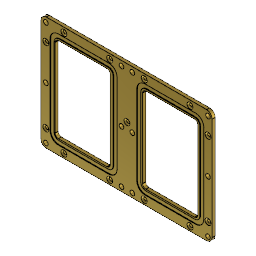
1006351A-exact-GASKET (Autodesk Fusion 360 design; units mm, degrees)
Autodesk Fusion 360 part; units mm, degrees
sketch "Front-OuterDimensionsAndHoles" plane through (0, 0, 0) normal (0, 1, 0) x (1, 0, 0) in component "1006351A-GASKET"
  line L0 (-137.0277, -51.6717) -> (147.7462, -51.6717) construction
  line L1 (-113.1932, -37.4477) -> (126.9355, -37.4477) construction
  line L2 (-111.6736, 46.3723) -> (88.9542, 46.3723) construction
  line L3 (-83.38, 4.4623) -> (113.9408, 4.4623) construction
  line L4 (77.012, -30.3357) -> (138.7437, -30.3357) construction
  line L5 (77.3795, 43.3243) -> (102.1824, 43.3243) construction
  line L6 (-79.2352, -152.4901) -> (-79.2352, 67.7682) construction
  line L7 (80.7848, -152.4901) -> (80.7848, 99.4049) construction
  line L8 (-16.2432, -127.3246) -> (-16.2432, -37.4477) construction
  line L9 (-61.4552, -139.7875) -> (-61.4552, -23.5467) construction
  line L10 (-4.5592, -114.8617) -> (-4.5592, -39.3651) construction
  line L11 (0.7748, -102.6384) -> (0.7748, 79.7518) construction
  line L12 (6.1088, -89.6961) -> (6.1088, 17.4372) construction
  line L13 (122.5447, -1.8877) -> (-114.7303, -1.8877) construction
  line L14 (151.0657, 56.0243) -> (-121.6808, 56.0243) construction
  line L15 (-84.366, -162.1054) -> (-84.366, 89.1529) construction
  line L16 (84.8488, -151.7017) -> (84.8488, 106.4269) construction
  line L17 (17.7928, -77.6983) -> (17.7928, -42.3651) construction
  line L18 (63.0048, -65.3317) -> (63.0048, -43.9355) construction
  line L19 (-137.1695, 60.5963) -> (174.7441, 60.5963) construction
  line L20 (-87.8994, -47.0997) -> (156.6849, -47.0997) construction
  line L21 (70.6248, 70.8097) -> (70.6248, -45.2683) construction
  line L22 (16.2688, 71.2679) -> (16.2688, -42.3651) construction
  line L23 (-15.786, 70.5042) -> (-15.786, -42.9773) construction
  line L24 (-70.142, 108.0768) -> (-70.142, -44.9628) construction
  line L25 (-10.9092, 93.2616) -> (-10.9092, -44.6574) construction
  line L26 (73.9383, 85.014) -> (73.9383, -42.8245) construction
  line L27 (-101.4005, 49.5796) -> (76.5348, 49.5796) construction
  line L28 (-100.0259, -41.454) -> (76.8403, -41.454) construction
  line L29 (-78.8288, -51.9257) -> (79.3116, -51.9257)
  line L30 (84.8488, -46.3885) -> (84.8488, 54.8051)
  line L31 (79.3116, 60.3423) -> (-78.8288, 60.3423)
  line L32 (-84.366, 54.8051) -> (-84.366, -46.3885)
  line L33 (-66.967, -37.7017) -> (-18.961, -37.7017)
  line L34 (-15.786, -34.5267) -> (-15.786, 42.9433)
  line L35 (-18.961, 46.1183) -> (-66.967, 46.1183)
  line L36 (-70.142, 42.9433) -> (-70.142, -34.5267)
  line L37 (19.4438, -37.7017) -> (67.4498, -37.7017)
  line L38 (70.6248, -34.5267) -> (70.6248, 42.9433)
  line L39 (67.4498, 46.1183) -> (19.4438, 46.1183)
  line L40 (16.2688, 42.9433) -> (16.2688, -34.5267)
  arc A0 (-84.366, -46.3885) -> (-78.8288, -51.9257) centre (-78.8288, -46.3885) ccw
  arc A1 (-78.8288, 60.3423) -> (-84.366, 54.8051) centre (-78.8288, 54.8051) ccw
  arc A2 (84.8488, 54.8051) -> (79.3116, 60.3423) centre (79.3116, 54.8051) ccw
  arc A3 (-70.142, -34.5267) -> (-66.967, -37.7017) centre (-66.967, -34.5267) ccw
  arc A4 (-18.961, -37.7017) -> (-15.786, -34.5267) centre (-18.961, -34.5267) ccw
  arc A5 (-15.786, 42.9433) -> (-18.961, 46.1183) centre (-18.961, 42.9433) ccw
  arc A6 (-66.967, 46.1183) -> (-70.142, 42.9433) centre (-66.967, 42.9433) ccw
  arc A7 (67.4498, -37.7017) -> (70.6248, -34.5267) centre (67.4498, -34.5267) ccw
  arc A8 (70.6248, 42.9433) -> (67.4498, 46.1183) centre (67.4498, 42.9433) ccw
  arc A9 (19.4438, 46.1183) -> (16.2688, 42.9433) centre (19.4438, 42.9433) ccw
  arc A10 (16.2688, -34.5267) -> (19.4438, -37.7017) centre (19.4438, -34.5267) ccw
  arc A11 (79.3116, -51.9257) -> (84.8488, -46.3885) centre (79.3116, -46.3885) ccw
  line L41 (-100.3246, -43.4352) -> (86.6573, -43.4352) construction
  line L42 (-99.9078, -39.4728) -> (77.154, -39.4728) construction
  line L43 (-94.8446, 47.5984) -> (76.1721, 47.5984) construction
  line L44 (-94.4522, 51.5608) -> (76.1721, 51.5608) construction
  line L45 (-73.1392, 86.7279) -> (-73.1392, -45.4577) construction
  line L46 (-8.928, 72.5566) -> (-8.928, -44.6167) construction
  line L47 (-12.8904, 72.2199) -> (-12.8904, -44.6167) construction
  line L48 (-75.1204, 70.9572) -> (-75.1204, -44.6167) construction
  line L49 (-71.158, 71.0414) -> (-71.158, -44.3641) construction
  line L50 (-66.967, 51.5608) -> (-17.0814, 51.5608)
  line L51 (-8.928, 43.4074) -> (-8.928, -35.2818)
  line L52 (-17.0814, -43.4352) -> (-66.967, -43.4352)
  line L53 (-75.1204, -35.2818) -> (-75.1204, 43.4074)
  line L54 (-66.205, 47.5984) -> (-17.8434, 47.5984)
  line L55 (-12.8904, 42.6454) -> (-12.8904, -34.5198)
  line L56 (-17.8434, -39.4728) -> (-66.205, -39.4728)
  line L57 (-71.158, -34.5198) -> (-71.158, 42.6454)
  arc A12 (-75.1204, -35.2818) -> (-66.967, -43.4352) centre (-66.967, -35.2818) ccw
  arc A13 (-17.0814, -43.4352) -> (-8.928, -35.2818) centre (-17.0814, -35.2818) ccw
  arc A14 (-8.928, 43.4074) -> (-17.0814, 51.5608) centre (-17.0814, 43.4074) ccw
  arc A15 (-66.967, 51.5608) -> (-75.1204, 43.4074) centre (-66.967, 43.4074) ccw
  arc A16 (-71.158, -34.5198) -> (-66.205, -39.4728) centre (-66.205, -34.5198) ccw
  arc A17 (-66.205, 47.5984) -> (-71.158, 42.6454) centre (-66.205, 42.6454) ccw
  arc A18 (-12.8904, 42.6454) -> (-17.8434, 47.5984) centre (-17.8434, 42.6454) ccw
  arc A19 (-17.8434, -39.4728) -> (-12.8904, -34.5198) centre (-17.8434, -34.5198) ccw
  line L58 (18.631, -43.4352) -> (68.5166, -43.4352)
  arc A20 (68.5166, -43.4352) -> (76.67, -35.2818) centre (68.5166, -35.2818) ccw
  line L59 (76.67, -35.2818) -> (76.67, 43.4074)
  arc A21 (76.67, 43.4074) -> (68.5166, 51.5608) centre (68.5166, 43.4074) ccw
  line L60 (68.5166, 51.5608) -> (18.631, 51.5608)
  arc A22 (18.631, 51.5608) -> (10.4776, 43.4074) centre (18.631, 43.4074) ccw
  line L61 (10.4776, 43.4074) -> (10.4776, -35.2818)
  arc A23 (10.4776, -35.2818) -> (18.631, -43.4352) centre (18.631, -35.2818) ccw
  line L62 (19.393, -39.4728) -> (67.7546, -39.4728)
  arc A24 (67.7546, -39.4728) -> (72.7076, -34.5198) centre (67.7546, -34.5198) ccw
  line L63 (72.7076, -34.5198) -> (72.7076, 42.6454)
  arc A25 (72.7076, 42.6454) -> (67.7546, 47.5984) centre (67.7546, 42.6454) ccw
  line L64 (67.7546, 47.5984) -> (19.393, 47.5984)
  arc A26 (19.393, 47.5984) -> (14.44, 42.6454) centre (19.393, 42.6454) ccw
  line L65 (14.44, 42.6454) -> (14.44, -34.5198)
  line L66 (101.4573, -39.4728) -> (-75.6045, -39.4728) construction
  arc A27 (14.44, -34.5198) -> (19.393, -39.4728) centre (19.393, -34.5198) ccw
  point P0 (-79.2352, -47.0997)
  point P1 (-4.5592, -47.0997)
  point P2 (6.1088, -47.0997)
  point P3 (80.7848, -47.0997)
  point P4 (80.7848, 4.4623)
  point P5 (6.1088, 4.4623)
  point P6 (-79.2352, 4.4623)
  point P7 (-4.5592, 4.4623)
  point P8 (80.7848, 56.0243)
  point P9 (6.1088, 56.0243)
  point P10 (-4.5592, 56.0243)
  point P11 (-79.2352, 56.0243)
  point P12 (80.7848, -30.3357)
  point P13 (80.7848, 43.3243)
  point P14 (63.0048, -47.0997)
  point P15 (17.7928, -47.0997)
  point P16 (17.7928, 56.0243)
  point P17 (63.0048, 56.0243)
  point P18 (0.7748, -1.8877)
  point P19 (-16.2432, -47.0997)
  point P20 (-61.4552, -47.0997)
  point P21 (-79.2352, -30.3357)
  point P22 (-79.2352, 43.3243)
  point P23 (-61.4552, 56.0243)
  point P24 (-16.2432, 56.0243)
  dimension "d1" = 169.2148
  dimension "d2" = 4.064
  dimension "d3" = 160.02
  dimension "d4" = 142.24
  dimension "d5" = 97.028
  dimension "d6" = 85.344
  dimension "d7" = 80.01
  dimension "d8" = 74.676
  dimension "d9" = 17.78
  dimension "d10" = 62.992
  dimension "d12" = 112.268
  dimension "d13" = 103.124
  dimension "d14" = 51.562
  dimension "d16" = 57.912
  dimension "d17" = 86.36
  dimension "d18" = 12.7
  dimension "d19" = 14.224
  dimension "d20" = 4.572
  dimension "d21" = 14.224
  dimension "d22" = 14.224
  dimension "d23" = 54.356
  dimension "d24" = 54.356
  dimension "d25" = 91.0336
  dimension "d26" = 14.224
  dimension "d27" = 5.5372
  dimension "d28" = 5.5372
  dimension "d29" = 5.5372
  dimension "d30" = 3.175
  dimension "d31" = 3.175
  dimension "d32" = 3.175
  dimension "d33" = 3.175
  dimension "d34" = 3.175
  dimension "d35" = 3.175
  dimension "d36" = 3.175
  dimension "d37" = 3.175
  dimension "d40" = 5.5372
  dimension "d49" = 1.9812
  dimension "d50" = 1.9812
  dimension "d51" = 1.9812
  dimension "d52" = 1.9812
  dimension "d53" = 91.694
  dimension "d54" = 62.23
  dimension "d55" = 1.9812
  dimension "d56" = 1.9812
  dimension "d57" = 1.9812
  dimension "d58" = 1.9812
  dimension "d59" = 8.1534
  dimension "d60" = 8.1534
  dimension "d61" = 8.1534
  dimension "d62" = 8.1534
  dimension "d63" = 4.953
  dimension "d64" = 4.953
  dimension "d65" = 4.953
  dimension "d66" = 4.953
  constraint horizontal L0
  constraint horizontal L1
  constraint parallel L1 L2
  constraint horizontal L3
  constraint parallel L1 L4
  constraint horizontal L5
  constraint perpendicular L0 L6
  constraint perpendicular L2 L7
  constraint coincident L1 L8.end
  constraint perpendicular L1 L8
  constraint vertical L9
  constraint perpendicular L0 L10
  constraint perpendicular L2 L11
  constraint perpendicular L3 L12
  constraint perpendicular L12 L13
  constraint parallel L2 L14
  constraint perpendicular L14 L15
  constraint perpendicular L14 L16
  constraint perpendicular L0 L17
  constraint perpendicular L0 L18
  constraint horizontal L19
  constraint perpendicular L15 L20
  constraint perpendicular L1 L21
  constraint perpendicular L1 L22
  constraint perpendicular L20 L23
  constraint perpendicular L1 L24
  constraint perpendicular L1 L25
  constraint perpendicular L1 L26
  constraint perpendicular L26 L27
  constraint perpendicular L26 L28
  constraint horizontal L29
  constraint vertical L30
  constraint horizontal L31
  constraint vertical L32
  constraint horizontal L33
  constraint vertical L34
  constraint horizontal L35
  constraint vertical L36
  constraint horizontal L37
  constraint vertical L38
  constraint horizontal L39
  constraint vertical L40
  constraint tangent L29 A0
  constraint tangent L32 A0
  constraint tangent L32 A1
  constraint tangent L31 A1
  constraint tangent L31 A2
  constraint tangent L30 A2
  constraint tangent L33 A3
  constraint tangent L36 A3
  constraint tangent L33 A4
  constraint tangent L34 A4
  constraint tangent L34 A5
  constraint tangent L35 A5
  constraint tangent L35 A6
  constraint tangent L36 A6
  constraint tangent L37 A7
  constraint tangent L38 A7
  constraint tangent L38 A8
  constraint tangent L39 A8
  constraint tangent L39 A9
  constraint tangent L40 A9
  constraint tangent L40 A10
  constraint tangent L37 A10
  constraint tangent L29 A11
  constraint tangent L30 A11
  constraint coincident L20 P0
  constraint coincident L6 P0
  constraint coincident L20 P1
  constraint coincident L10 P1
  constraint coincident L12 P2
  constraint coincident L20 P2
  constraint coincident L20 P3
  constraint coincident L7 P3
  constraint coincident L3 P4
  constraint coincident L7 P4
  constraint coincident L12 P5
  constraint coincident L3 P5
  constraint symmetric L11 P4 P6
  constraint symmetric L11 P5 P7
  constraint symmetric L3 P0 P11
  constraint symmetric L3 P1 P10
  constraint symmetric L3 P2 P9
  constraint symmetric L3 P3 P8
  constraint coincident L4 P12
  constraint coincident L7 P12
  constraint coincident L7 P13
  constraint coincident L5 P13
  constraint coincident L18 P14
  constraint coincident L20 P14
  constraint coincident L17 P15
  constraint coincident L20 P15
  constraint symmetric L3 P14 P17
  constraint symmetric L3 P15 P16
  constraint coincident L13 P18
  constraint coincident L11 P18
  constraint symmetric L11 P12 P21
  constraint symmetric L11 P13 P22
  constraint symmetric L11 P14 P20
  constraint symmetric L11 P15 P19
  constraint symmetric L11 P16 P24
  constraint symmetric L11 P17 P23
  constraint parallel L28 L41
  constraint perpendicular L12 L42
  constraint parallel L27 L43
  constraint perpendicular L22 L44
  constraint perpendicular L20 L45
  constraint perpendicular L41 L46
  constraint perpendicular L41 L47
  constraint perpendicular L41 L48
  constraint perpendicular L41 L49
  constraint horizontal L50
  constraint vertical L51
  constraint horizontal L52
  constraint vertical L53
  constraint horizontal L54
  constraint vertical L55
  constraint horizontal L56
  constraint vertical L57
  constraint tangent L52 A12
  constraint tangent L53 A12
  constraint tangent L52 A13
  constraint tangent L51 A13
  constraint tangent L51 A14
  constraint tangent L50 A14
  constraint tangent L50 A15
  constraint tangent L53 A15
  constraint tangent L56 A16
  constraint tangent L57 A16
  constraint tangent L57 A17
  constraint tangent L54 A17
  constraint tangent L54 A18
  constraint tangent L55 A18
  constraint tangent L55 A19
  constraint tangent L56 A19
  constraint symmetric L11 L42.start L66.start
  constraint symmetric L11 L42.end L66.end
  constraint symmetric L11 L52.end L58.end
  constraint symmetric L11 L53.start A20.end
  constraint symmetric L11 A12 A20
  constraint symmetric L11 L52.start L58.start
  constraint symmetric L11 L51.end L61.end
  constraint symmetric L11 A13 A23
  constraint symmetric L11 L51.start A22.end
  constraint symmetric L11 L50.end L60.end
  constraint symmetric L11 A14 A22
  constraint symmetric L11 L50.start A21.end
  constraint symmetric L11 L53.end L59.end
  constraint symmetric L11 A15 A21
  constraint symmetric L11 L56.end L62.end
  constraint symmetric L11 L57.start A24.end
  constraint symmetric L11 A16 A24
  constraint symmetric L11 L57.end L63.end
  constraint symmetric L11 L54.start A25.end
  constraint symmetric L11 A17 A25
  constraint symmetric L11 L54.end L64.end
  constraint symmetric L11 L55.start A26.end
  constraint symmetric L11 A18 A26
  constraint symmetric L11 L55.end L65.end
  constraint symmetric L11 L56.start L62.start
  constraint symmetric L11 A19 A27
  measures "d1" distance of L15 L16
  measures "d2" distance of L7 L16
  measures "d3" distance of L6 L7
  measures "d4" distance of L7 L9
  measures "d5" distance of L7 L8
  measures "d6" distance of L7 L10
  measures "d7" distance of L7 L11
  measures "d8" distance of L7 L12
  measures "d9" distance of L7 L18
  measures "d10" distance of L7 L17
  measures "d12" distance of L0 L19
  measures "d13" distance of L14 L20
  measures "d14" distance of L3 L14
  measures "d16" distance of L13 L14
  measures "d17" distance of L4 L14
  measures "d18" distance of L5 L14
  measures "d19" distance of L2 L19
  measures "d20" distance of L14 L19
  measures "d21" distance of L0 L1
  measures "d22" distance of L16 L21
  measures "d23" distance of L21 L22
  measures "d24" distance of L23 L24
  measures "d25" distance of L27 L28
  measures "d26" distance of L15 L24
  measures "d27" radius of A0
  measures "d28" radius of A1
  measures "d29" radius of A2
  measures "d30" radius of A3
  measures "d31" radius of A4
  measures "d32" radius of A5
  measures "d33" radius of A6
  measures "d34" radius of A7
  measures "d35" radius of A8
  measures "d36" radius of A9
  measures "d37" radius of A10
  measures "d40" radius of A11
  measures "d49" distance of L28 L41
  measures "d50" distance of L28 L42
  measures "d51" distance of L27 L43
  measures "d52" distance of L27 L44
  measures "d53" distance of L7 L25
  measures "d54" distance of L25 L45
  measures "d55" distance of L25 L46
  measures "d56" distance of L25 L47
  measures "d57" distance of L45 L48
  measures "d58" distance of L45 L49
  measures "d59" radius of A12
  measures "d60" radius of A13
  measures "d61" radius of A14
  measures "d62" radius of A15
  measures "d63" radius of A16
  measures "d64" radius of A17
  measures "d65" radius of A18
  measures "d66" radius of A19
extrude "Extrude1" add sketch "Front-OuterDimensionsAndHoles" along normal blind 3.2004 contours L29 L30 L31 L32 A0 A1 A2 A11 | L50 L51 L52 L53 A12 A13 A14 A15 | L54 L55 L56 L57 A16 A17 A18 A19 | L58 A20 L59 A21 L60 A22 L61 A23 | L62 A24 L63 A25 L64 A26 L65 A27 in component "1006351A-GASKET"
hole "Hole1" at (80.7848, 0, 47.0997) at (6.1088, 0, 47.0997) at (-4.5592, 0, 47.0997) at (-79.2352, 0, 47.0997) at (-79.2352, 0, -56.0243) at (6.1088, 0, -56.0243) at (-4.5592, 0, -56.0243) at (80.7848, 0, -56.0243) at (80.7848, 0, -4.4623) at (6.1088, 0, -4.4623) at (-4.5592, 0, -4.4623) at (-79.2352, 0, -4.4623) direction (0, 1, 0) diameter 4.572 end through all in component "1006351A-GASKET"
hole "Hole2" at (-61.4552, 0, 47.0997) at (-16.2432, 0, 47.0997) at (17.7928, 0, 47.0997) at (63.0048, 0, 47.0997) at (80.7848, 0, 30.3357) at (80.7848, 0, -43.3243) at (63.0048, 0, -56.0243) at (0.7748, 0, 1.8877) at (-16.2432, 0, -56.0243) at (17.7928, 0, -56.0243) at (-61.4552, 0, -56.0243) at (-79.2352, 0, -43.3243) at (-79.2352, 0, 30.3357) direction (0, 1, 0) diameter 3.3782 end through all countersink diameter 5.842 countersink angle 82 in component "1006351A-GASKET"
extrude "Extrude2" cut sketch "Front-OuterDimensionsAndHoles" along normal blind 0.6604 contours L50 L51 L52 L53 A12 A13 A14 A15 | L58 A20 L59 A21 L60 A22 L61 A23 in component "1006351A-GASKET"
component "1006351A-GASKET" placed x (1, 0, 0) y (0, 1, 0) z (0, 0, 1) at (0, 0, 0)
equation "d49 = ( 0.156 / 2 ) * 1 in"
equation "d50 = ( 0.156 / 2 ) * 1 in"
equation "d51 = ( 0.156 / 2 ) * 1 in"
equation "d52 = ( 0.156 / 2 ) * 1 in"
